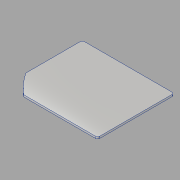
# Autodesk Inventor part: Base Plate Mk 2
Saved by Autodesk Inventor 2017 (Build 210142000, 142)
## iProperties
Created: 2016-12-06
Part Number: Base Plate Mk 2
Material: Aluminum 6061
Document SubType Name: Modeling
Designer: qupec
Density: 2.7 g/cm^3
Appearance: Aluminum - Flat
Author: qupec
Autodesk Inventor part; units mm, degrees
ref_plane "YZ Plane" through (0, 0, 0) normal (1, 0, 0) x (0, 1, 0)
ref_plane "XZ Plane" through (0, 0, 0) normal (0, 1, 0) x (-1, 0, 0)
ref_plane "XY Plane" through (0, 0, 0) normal (0, 0, 1) x (1, 0, 0)
sketch "Sketch1" plane through (0, 0, 0) normal (0, 1, 0) x (-1, 0, 0)
  line L0 (76.2, 63.5) -> (-76.2, 63.5)
  line L1 (-76.2, 63.5) -> (-76.2, -63.5)
  line L2 (-76.2, -63.5) -> (76.2, -63.5)
  line L3 (76.2, -63.5) -> (76.2, 63.5)
  point P0 (0, 0)
  dimension "d0" = 127
  dimension "d1" = 152.4
  dimension "d2" = 76.2
  dimension "d3" = 63.5
  constraints: 8 end point, 2 parallel, 1 horizontal, 1 perpendicular
  measures "d0" distance of L2.end L0.start
  measures "d1" distance of L0.start L0.end
  measures "d2" distance from line of point (0, 0) L1
  measures "d3" distance from line of point (0, 0) L0
extrude "Extrusion1" add sketch "Sketch1" along normal blind 3.175
sketch "Sketch4" plane through (0, 3.175, 0) normal (0, 1, 0) x (1, 0, 0)
  circle A0 centre (69.85, 57.15) radius 3.175
  circle A1 centre (69.85, -57.15) radius 3.175
  circle A2 centre (-67.31, -39.37) radius 3.175
  line L0 (76.2, 63.5) -> (-76.2, 63.5) projected
  line L1 (76.2, -63.5) -> (76.2, 63.5) projected
  line L2 (-76.2, -63.5) -> (76.2, -63.5) projected
  line L3 (-76.2, 63.5) -> (-76.2, -63.5) projected
  circle A3 centre (-67.31, 39.37) radius 3.175
  point P0 (0, 0)
  dimension "d20" = 6.35
  dimension "d21" = 6.35
  dimension "d22" = 6.35
  dimension "d23" = 6.35
  dimension "d24" = 6.35
  dimension "d25" = 6.35
  dimension "d26" = 6.35
  dimension "d27" = 24.13
  dimension "d28" = 8.89
  dimension "d32" = 6.35
  dimension "d33" = 24.13
  dimension "d34" = 8.89
  constraints: 4 centre point
  measures "d20" diameter of A2
  measures "d21" diameter of A1
  measures "d22" diameter of A0
  measures "d23" distance from line of L0 A0.centre
  measures "d24" distance from line of L1 A0.centre
  measures "d25" distance from line of L1 A1.centre
  measures "d26" distance from line of L2 A1.centre
  measures "d27" distance from line of L2 A2.centre
  measures "d28" distance from line of L3 A2.centre
  measures "d32" diameter of A3
  measures "d33" distance from line of L0 A3.centre
  measures "d34" distance from line of L3 A3.centre
extrude "Extrusion6" [suppressed]
fillet "Fillet1" radius 3.175 4 edges at (-76.2, 1.5875, 63.5) (76.2, 1.5875, 63.5) (76.2, 1.5875, -63.5) (-76.2, 1.5875, -63.5)
sketch "Sketch7" plane through (0, 3.175, 0) normal (0, 1, 0) x (1, 0, 0)
  circle A0 centre (50.8, 53.8226) radius 152.4
  line L0 (73.025, 63.5) -> (-73.025, 63.5) projected
  line L1 (76.2, -60.325) -> (76.2, 60.325) projected
  arc A1 (-76.2, -60.325) -> (-73.025, -63.5) centre (-73.025, -60.325) ccw projected
  line L2 (-73.025, -63.5) -> (73.025, -63.5) projected
  line L3 (-73.025, -63.5) -> (-46.4685, -63.5)
  line L4 (-76.2, 60.325) -> (-76.2, -60.325) projected
  line L5 (-76.2, -60.325) -> (-76.2, -30.4197)
  point P0 (0, 0)
  point P1 (73.025, -60.325)
  point P2 (73.025, 60.325)
  dimension "d46" = 304.8
  dimension "d47" = 9.6774
  dimension "d48" = 25.4
  constraints: 4 end point, 3 point on line, 2 point on circle, 1 centre point
  measures "d46" diameter of A0
  measures "d47" distance from line of L0 A0.centre
  measures "d48" distance from line of L1 A0.centre
extrude "Extrusion8" cut sketch "Sketch7" against normal through all contours A0 L2 A1 L4
equation "\"d2\" = 0.5 * d1"
equation "\"d3\" = 0.5 * d0"
equation "\"d21\" = d20"
equation "\"d22\" = d20"
equation "\"d24\" = d23"
equation "\"d25\" = d24"
equation "\"d26\" = d23"
equation "\"d32\" = d20"
equation "\"d33\" = d27"
equation "\"d34\" = d28"
body "Solid1"
